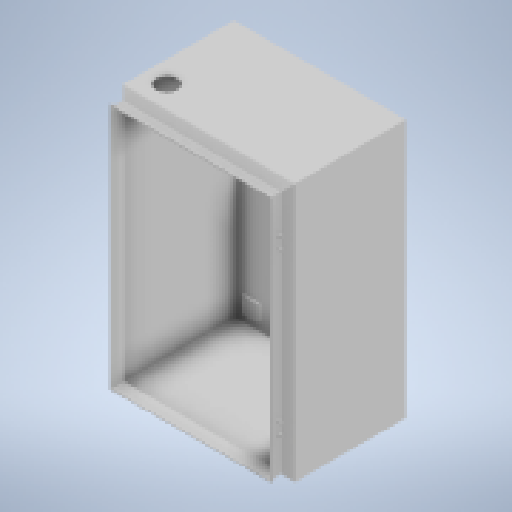
# Autodesk Inventor part: 1301.000_1_(1)
Saved by Autodesk Inventor 2025.2 (Build 292293000, 293)
## iProperties
Category: PARTsolutions
Company: RITTAL
Created: 2025-05-02
Part Number: 1301.000_1_(1)
Material: Generic
Catalog Web Link: www.cadenas.de
Description: Gehaeuse KX EB Edelstahl-Gehaeuse KX EB Edelstahl
Vendor: RITTAL
Document SubType Name: Modeling
Designer: psAdmin
Manufacturer: RITTAL
Mass: 264.521 g
Surface Area: 4243.67 cm^2
Volume: 264.521 cm^3
Density: 1 g/cm^3
Appearance: PSOLRGB-175-175-175
PSOL_IDENT_0: {$CADENAS_DATA/23d-libs/rittal/schaltschranksys/edelstahl/kleingehause/parts_eb_edel_2_0/gehaeuse_kx
PSOL_IDENT_1: _eb_edel_new.prj},199 {VTYP=3D},{NB=1301.000_1_(1)},{LINA=1301.000_1_(1)},{NN=Gehaeuse KX EB Edelsta
PSOL_IDENT_2: hl},{DATE=28.04.2025 21:10:48},{GEOMDATE=11.04.2025 11:21:29},{VERSION=},{LINEID=690},{WBVAR=DETAIL}
PSOL_IDENT_3: ,{WBNUMERIC=DETAIL}  {NB=1301.000_1_(1)},{LINA=1301.000_1_(1)},{KT=DUMMY},{BEST=1301.000},{S=1.25},{
PSOL_IDENT_4: DETAIL=1},{B1=200},{H1=300},{T1=152.750},{B2=160.000},{B3=187},{L=133},{L1=75},{N=6},{H2=260},{T=155
PSOL_IDENT_5: .000},{GEW=3,889},{T2=130.000},{CNSETIM80=EC000261},{CNSETIM90=EC000261},{CNSECLASS60=27-18-01-01},{
PSOL_IDENT_6: CNSECLASS80=27-18-01-01},{UNSPSC=31-26-15-02}
NB: 1301.000_1_(1)
NN: Gehaeuse KX EB Edelstahl
NT: Gehaeuse KX EB Edelstahl
NBSYN: $BEST._1_($DETAIL.)
LINA: 1301.000_1_(1)
CATALOG: Rittal
BEST: 1301.000
S: 1.25
DETAIL: hoch
B1: 200
H1: 300
T1: 152.75
B2: 160
B3: 187
L: 133
L1: 75
N: 6
H2: 260
T: 155
GEW: 3,889
T2: 130
CNSETIM80: EC000261
CNSETIM90: EC000261
CNSECLASS60: 27-18-01-01
CNSECLASS80: 27-18-01-01
UNSPSC: 31-26-15-02
SUPPLIER: RITTAL
ARTICLENO: 1301.000_1_(1)
BOMINFO: 1301.000_1_(1)
CREATOR: CADENAS GmbH
Title: 1301.000_1_(1)
Author: Cadenas PARTsolutions
Comments: Gehaeuse KX EB Edelstahl
Autodesk Inventor part; units mm, degrees
(part 1 of 2)
ref_plane "YZ Plane" through (0, 0, 0) normal (1, 0, 0) x (0, 1, 0)
ref_plane "XZ Plane" through (0, 0, 0) normal (0, 1, 0) x (-1, 0, 0)
ref_plane "XY Plane" through (0, 0, 0) normal (0, 0, 1) x (1, 0, 0)
sketch "Skizze_2" plane through (0, 0, 0) normal (1, 0, 0) x (0, 0, -1)
  line L0 (-75.4448, -142.2749) -> (-75.1213, -143.4823)
  line L1 (-75.1213, -143.4823) -> (-69.0017, -141.8426)
  arc A0 (-68.6782, -141.8) -> (-69.0017, -141.8426) centre (-68.6782, -143.05) ccw
  line L2 (-68.6782, -141.8) -> (-62.8605, -141.8)
  arc A1 (-61.9767, -142.1661) -> (-62.8605, -141.8) centre (-62.8605, -143.05) ccw
  line L3 (-61.9767, -142.1661) -> (-54.875, -149.2678)
  arc A2 (-54.875, -149.2678) -> (-53.1072, -150) centre (-53.1072, -147.5) ccw
  line L4 (-53.1072, -150) -> (76.375, -150)
  line L5 (76.375, -150) -> (76.375, 150)
  line L6 (76.375, 150) -> (-53.1072, 150)
  arc A3 (-53.1072, 150) -> (-54.875, 149.2678) centre (-53.1072, 147.5) ccw
  line L7 (-54.875, 149.2678) -> (-61.9767, 142.1661)
  arc A4 (-62.8605, 141.8) -> (-61.9767, 142.1661) centre (-62.8605, 143.05) ccw
  line L8 (-62.8605, 141.8) -> (-68.6782, 141.8)
  arc A5 (-69.0017, 141.8426) -> (-68.6782, 141.8) centre (-68.6782, 143.05) ccw
  line L9 (-69.0017, 141.8426) -> (-75.1213, 143.4823)
  line L10 (-75.1213, 143.4823) -> (-75.4448, 142.2749)
  line L11 (-75.4448, 142.2749) -> (-69.3252, 140.6352)
  arc A6 (-69.3252, 140.6352) -> (-68.6782, 140.55) centre (-68.6782, 143.05) ccw
  line L12 (-68.6782, 140.55) -> (-62.8605, 140.55)
  arc A7 (-62.8605, 140.55) -> (-61.0928, 141.2822) centre (-62.8605, 143.05) ccw
  line L13 (-61.0928, 141.2822) -> (-53.9911, 148.3839)
  arc A8 (-53.1072, 148.75) -> (-53.9911, 148.3839) centre (-53.1072, 147.5) ccw
  line L14 (-53.1072, 148.75) -> (73.875, 148.75)
  arc A9 (75.125, 147.5) -> (73.875, 148.75) centre (73.875, 147.5) ccw
  line L15 (75.125, 147.5) -> (75.125, -147.5)
  arc A10 (73.875, -148.75) -> (75.125, -147.5) centre (73.875, -147.5) ccw
  line L16 (73.875, -148.75) -> (-53.1072, -148.75)
  arc A11 (-53.9911, -148.3839) -> (-53.1072, -148.75) centre (-53.1072, -147.5) ccw
  line L17 (-53.9911, -148.3839) -> (-61.0928, -141.2822)
  arc A12 (-61.0928, -141.2822) -> (-62.8605, -140.55) centre (-62.8605, -143.05) ccw
  line L18 (-62.8605, -140.55) -> (-68.6782, -140.55)
  arc A13 (-68.6782, -140.55) -> (-69.3252, -140.6352) centre (-68.6782, -143.05) ccw
  line L19 (-69.3252, -140.6352) -> (-75.4448, -142.2749)
  constraints: 40 end point, 28 point on circle, 14 centre point
extrude "Extrusion1" add sketch "Skizze_2" along normal mid plane 200
sketch "Sketch_1" plane through (0, 0, 0) normal (0, 1, 0) x (-1, 0, 0)
  line L0 (100, -76.375) -> (100, 53.1072)
  arc A0 (100, 53.1072) -> (99.2678, 54.875) centre (97.5, 53.1072) ccw
  line L1 (99.2678, 54.875) -> (92.1661, 61.9767)
  arc A1 (91.8, 62.8605) -> (92.1661, 61.9767) centre (93.05, 62.8605) ccw
  line L2 (91.8, 62.8605) -> (91.8, 68.6782)
  arc A2 (91.8426, 69.0017) -> (91.8, 68.6782) centre (93.05, 68.6782) ccw
  line L3 (91.8426, 69.0017) -> (93.4823, 75.1213)
  line L4 (93.4823, 75.1213) -> (92.2749, 75.4448)
  line L5 (92.2749, 75.4448) -> (90.6352, 69.3252)
  arc A3 (90.6352, 69.3252) -> (90.55, 68.6782) centre (93.05, 68.6782) ccw
  line L6 (90.55, 68.6782) -> (90.55, 62.8605)
  arc A4 (90.55, 62.8605) -> (91.2822, 61.0928) centre (93.05, 62.8605) ccw
  line L7 (91.2822, 61.0928) -> (98.3839, 53.9911)
  arc A5 (98.75, 53.1072) -> (98.3839, 53.9911) centre (97.5, 53.1072) ccw
  line L8 (98.75, 53.1072) -> (98.75, -73.875)
  arc A6 (97.5, -75.125) -> (98.75, -73.875) centre (97.5, -73.875) ccw
  line L9 (97.5, -75.125) -> (-97.5, -75.125)
  arc A7 (-98.75, -73.875) -> (-97.5, -75.125) centre (-97.5, -73.875) ccw
  line L10 (-98.75, -73.875) -> (-98.75, 53.1072)
  arc A8 (-98.3839, 53.9911) -> (-98.75, 53.1072) centre (-97.5, 53.1072) ccw
  line L11 (-98.3839, 53.9911) -> (-91.2822, 61.0928)
  arc A9 (-91.2822, 61.0928) -> (-90.55, 62.8605) centre (-93.05, 62.8605) ccw
  line L12 (-90.55, 62.8605) -> (-90.55, 68.6782)
  arc A10 (-90.55, 68.6782) -> (-90.6352, 69.3252) centre (-93.05, 68.6782) ccw
  line L13 (-90.6352, 69.3252) -> (-92.2749, 75.4448)
  line L14 (-92.2749, 75.4448) -> (-93.4823, 75.1213)
  line L15 (-93.4823, 75.1213) -> (-91.8426, 69.0017)
  arc A11 (-91.8, 68.6782) -> (-91.8426, 69.0017) centre (-93.05, 68.6782) ccw
  line L16 (-91.8, 68.6782) -> (-91.8, 62.8605)
  arc A12 (-92.1661, 61.9767) -> (-91.8, 62.8605) centre (-93.05, 62.8605) ccw
  line L17 (-92.1661, 61.9767) -> (-99.2678, 54.875)
  arc A13 (-99.2678, 54.875) -> (-100, 53.1072) centre (-97.5, 53.1072) ccw
  line L18 (-100, 53.1072) -> (-100, -76.375)
  line L19 (-100, -76.375) -> (100, -76.375)
  constraints: 40 end point, 28 point on circle, 14 centre point
extrude "Extrusion2" add sketch "Sketch_1" along normal mid plane 300
sketch "Sketch_37" plane through (0, 0, 0) normal (1, 0, 0) x (0, 0, -1)
  line L0 (-86.375, -160) -> (86.375, -160)
  line L1 (86.375, -160) -> (86.375, 160)
  line L2 (86.375, 160) -> (-86.375, 160)
  line L3 (-86.375, 160) -> (-86.375, -160)
  line L4 (-75.4448, -142.2749) -> (-75.1213, -143.4823)
  line L5 (-75.1213, -143.4823) -> (-69.0017, -141.8426)
  arc A0 (-68.6782, -141.8) -> (-69.0017, -141.8426) centre (-68.6782, -143.05) ccw
  line L6 (-68.6782, -141.8) -> (-62.8605, -141.8)
  arc A1 (-61.9767, -142.1661) -> (-62.8605, -141.8) centre (-62.8605, -143.05) ccw
  line L7 (-61.9767, -142.1661) -> (-54.875, -149.2678)
  arc A2 (-54.875, -149.2678) -> (-53.1072, -150) centre (-53.1072, -147.5) ccw
  line L8 (-53.1072, -150) -> (73.875, -150)
  arc A3 (73.875, -150) -> (76.375, -147.5) centre (73.875, -147.5) ccw
  line L9 (76.375, -147.5) -> (76.375, 147.5)
  arc A4 (76.375, 147.5) -> (73.875, 150) centre (73.875, 147.5) ccw
  line L10 (73.875, 150) -> (-53.1072, 150)
  arc A5 (-53.1072, 150) -> (-54.875, 149.2678) centre (-53.1072, 147.5) ccw
  line L11 (-54.875, 149.2678) -> (-61.9767, 142.1661)
  arc A6 (-62.8605, 141.8) -> (-61.9767, 142.1661) centre (-62.8605, 143.05) ccw
  line L12 (-62.8605, 141.8) -> (-68.6782, 141.8)
  arc A7 (-69.0017, 141.8426) -> (-68.6782, 141.8) centre (-68.6782, 143.05) ccw
  line L13 (-69.0017, 141.8426) -> (-75.1213, 143.4823)
  line L14 (-75.1213, 143.4823) -> (-75.4448, 142.2749)
  line L15 (-75.4448, 142.2749) -> (-75.4448, -142.2749)
  constraints: 32 end point, 16 point on circle, 8 centre point
extrude "Extrusion3" cut sketch "Sketch_37" along normal mid plane 200
sketch "Sketch_38" plane through (0, 0, 0) normal (0, 1, 0) x (-1, 0, 0)
  line L0 (110, 86.375) -> (-110, 86.375)
  line L1 (-110, 86.375) -> (-110, -86.375)
  line L2 (-110, -86.375) -> (110, -86.375)
  line L3 (110, -86.375) -> (110, 86.375)
  line L4 (100, -73.875) -> (100, 53.1072)
  arc A0 (100, 53.1072) -> (99.2678, 54.875) centre (97.5, 53.1072) ccw
  line L5 (99.2678, 54.875) -> (92.1661, 61.9767)
  arc A1 (91.8, 62.8605) -> (92.1661, 61.9767) centre (93.05, 62.8605) ccw
  line L6 (91.8, 62.8605) -> (91.8, 68.6782)
  arc A2 (91.8426, 69.0017) -> (91.8, 68.6782) centre (93.05, 68.6782) ccw
  line L7 (91.8426, 69.0017) -> (93.4823, 75.1213)
  line L8 (93.4823, 75.1213) -> (92.2749, 75.4448)
  line L9 (92.2749, 75.4448) -> (-92.2749, 75.4448)
  line L10 (-92.2749, 75.4448) -> (-93.4823, 75.1213)
  line L11 (-93.4823, 75.1213) -> (-91.8426, 69.0017)
  arc A3 (-91.8, 68.6782) -> (-91.8426, 69.0017) centre (-93.05, 68.6782) ccw
  line L12 (-91.8, 68.6782) -> (-91.8, 62.8605)
  arc A4 (-92.1661, 61.9767) -> (-91.8, 62.8605) centre (-93.05, 62.8605) ccw
  line L13 (-92.1661, 61.9767) -> (-99.2678, 54.875)
  arc A5 (-99.2678, 54.875) -> (-100, 53.1072) centre (-97.5, 53.1072) ccw
  line L14 (-100, 53.1072) -> (-100, -73.875)
  arc A6 (-100, -73.875) -> (-97.5, -76.375) centre (-97.5, -73.875) ccw
  line L15 (-97.5, -76.375) -> (97.5, -76.375)
  arc A7 (97.5, -76.375) -> (100, -73.875) centre (97.5, -73.875) ccw
  constraints: 32 end point, 16 point on circle, 8 centre point
extrude "Extrusion4" cut sketch "Sketch_38" along normal mid plane 300
sketch "Sketch_2" plane through (0, 0, -76.375) normal (0, 0, 1) x (1, 0, 0)
  line L0 (67.5, 142.5) -> (67.5, 117.5)
  line L1 (67.5, 117.5) -> (92.5, 117.5)
  line L2 (92.5, 117.5) -> (92.5, 142.5)
  line L3 (92.5, 142.5) -> (67.5, 142.5)
  constraints: 8 end point
extrude "Extrusion5" cut sketch "Sketch_2" along normal blind 3.25
sketch "Sketch_9" plane through (0, 0, -76.375) normal (0, 0, 1) x (1, 0, 0)
  line L0 (-92.5, 142.5) -> (-92.5, 117.5)
  line L1 (-92.5, 117.5) -> (-67.5, 117.5)
  line L2 (-67.5, 117.5) -> (-67.5, 142.5)
  line L3 (-67.5, 142.5) -> (-92.5, 142.5)
  constraints: 8 end point
extrude "Extrusion6" cut sketch "Sketch_9" along normal blind 3.25
sketch "Sketch_10" plane through (0, 0, -76.375) normal (0, 0, 1) x (1, 0, 0)
  line L0 (67.5, -117.5) -> (67.5, -142.5)
  line L1 (67.5, -142.5) -> (92.5, -142.5)
  line L2 (92.5, -142.5) -> (92.5, -117.5)
  line L3 (92.5, -117.5) -> (67.5, -117.5)
  constraints: 8 end point
extrude "Extrusion7" cut sketch "Sketch_10" along normal blind 3.25
sketch "Sketch_11" plane through (0, 0, -76.375) normal (0, 0, 1) x (1, 0, 0)
  line L0 (-92.5, -117.5) -> (-92.5, -142.5)
  line L1 (-92.5, -142.5) -> (-67.5, -142.5)
  line L2 (-67.5, -142.5) -> (-67.5, -117.5)
  line L3 (-67.5, -117.5) -> (-92.5, -117.5)
  constraints: 8 end point
extrude "Extrusion8" cut sketch "Sketch_11" along normal blind 3.25
sketch "Sketch_30" plane through (0, 130, 0) normal (0, 1, 0) x (1, 0, 0)
  line L0 (66.5, 75.125) -> (69.0034, 75.125)
  arc A0 (69.2528, 74.9917) -> (69.0034, 75.125) centre (69.0034, 74.825) ccw
  line L1 (69.2528, 74.9917) -> (70.0546, 73.7917)
  arc A1 (70.0546, 73.7917) -> (71.3018, 73.125) centre (71.3018, 74.625) ccw
  line L2 (71.3018, 73.125) -> (88.6982, 73.125)
  arc A2 (88.6982, 73.125) -> (89.9454, 73.7917) centre (88.6982, 74.625) ccw
  line L3 (89.9454, 73.7917) -> (90.7472, 74.9917)
  arc A3 (90.9966, 75.125) -> (90.7472, 74.9917) centre (90.9966, 74.825) ccw
  line L4 (90.9966, 75.125) -> (93.5, 75.125)
  line L5 (93.5, 75.125) -> (93.5, 76.375)
  line L6 (93.5, 76.375) -> (90.9699, 76.375)
  arc A4 (90.9699, 76.375) -> (89.7227, 75.7083) centre (90.9699, 74.875) ccw
  line L7 (89.7227, 75.7083) -> (88.9209, 74.5083)
  arc A5 (88.6715, 74.375) -> (88.9209, 74.5083) centre (88.6715, 74.675) ccw
  line L8 (88.6715, 74.375) -> (71.3285, 74.375)
  arc A6 (71.0791, 74.5083) -> (71.3285, 74.375) centre (71.3285, 74.675) ccw
  line L9 (71.0791, 74.5083) -> (70.2773, 75.7083)
  arc A7 (70.2773, 75.7083) -> (69.0301, 76.375) centre (69.0301, 74.875) ccw
  line L10 (69.0301, 76.375) -> (66.5, 76.375)
  line L11 (66.5, 76.375) -> (66.5, 75.125)
  constraints: 24 end point, 16 point on circle, 8 centre point
extrude "Extrusion9" add sketch "Sketch_30" along normal mid plane 15.297
sketch "Sketch_31" plane through (0, 130, 0) normal (0, 1, 0) x (1, 0, 0)
  line L0 (-93.5, 75.125) -> (-90.9966, 75.125)
  arc A0 (-90.7472, 74.9917) -> (-90.9966, 75.125) centre (-90.9966, 74.825) ccw
  line L1 (-90.7472, 74.9917) -> (-89.9454, 73.7917)
  arc A1 (-89.9454, 73.7917) -> (-88.6982, 73.125) centre (-88.6982, 74.625) ccw
  line L2 (-88.6982, 73.125) -> (-71.3018, 73.125)
  arc A2 (-71.3018, 73.125) -> (-70.0546, 73.7917) centre (-71.3018, 74.625) ccw
  line L3 (-70.0546, 73.7917) -> (-69.2528, 74.9917)
  arc A3 (-69.0034, 75.125) -> (-69.2528, 74.9917) centre (-69.0034, 74.825) ccw
  line L4 (-69.0034, 75.125) -> (-66.5, 75.125)
  line L5 (-66.5, 75.125) -> (-66.5, 76.375)
  line L6 (-66.5, 76.375) -> (-69.0301, 76.375)
  arc A4 (-69.0301, 76.375) -> (-70.2773, 75.7083) centre (-69.0301, 74.875) ccw
  line L7 (-70.2773, 75.7083) -> (-71.0791, 74.5083)
  arc A5 (-71.3285, 74.375) -> (-71.0791, 74.5083) centre (-71.3285, 74.675) ccw
  line L8 (-71.3285, 74.375) -> (-88.6715, 74.375)
  arc A6 (-88.9209, 74.5083) -> (-88.6715, 74.375) centre (-88.6715, 74.675) ccw
  line L9 (-88.9209, 74.5083) -> (-89.7227, 75.7083)
  arc A7 (-89.7227, 75.7083) -> (-90.9699, 76.375) centre (-90.9699, 74.875) ccw
  line L10 (-90.9699, 76.375) -> (-93.5, 76.375)
  line L11 (-93.5, 76.375) -> (-93.5, 75.125)
  constraints: 24 end point, 16 point on circle, 8 centre point
extrude "Extrusion10" add sketch "Sketch_31" along normal mid plane 15.297
sketch "Sketch_32" plane through (0, -130, 0) normal (0, 1, 0) x (1, 0, 0)
  line L0 (66.5, 75.125) -> (69.0034, 75.125)
  arc A0 (69.2528, 74.9917) -> (69.0034, 75.125) centre (69.0034, 74.825) ccw
  line L1 (69.2528, 74.9917) -> (70.0546, 73.7917)
  arc A1 (70.0546, 73.7917) -> (71.3018, 73.125) centre (71.3018, 74.625) ccw
  line L2 (71.3018, 73.125) -> (88.6982, 73.125)
  arc A2 (88.6982, 73.125) -> (89.9454, 73.7917) centre (88.6982, 74.625) ccw
  line L3 (89.9454, 73.7917) -> (90.7472, 74.9917)
  arc A3 (90.9966, 75.125) -> (90.7472, 74.9917) centre (90.9966, 74.825) ccw
  line L4 (90.9966, 75.125) -> (93.5, 75.125)
  line L5 (93.5, 75.125) -> (93.5, 76.375)
  line L6 (93.5, 76.375) -> (90.9699, 76.375)
  arc A4 (90.9699, 76.375) -> (89.7227, 75.7083) centre (90.9699, 74.875) ccw
  line L7 (89.7227, 75.7083) -> (88.9209, 74.5083)
  arc A5 (88.6715, 74.375) -> (88.9209, 74.5083) centre (88.6715, 74.675) ccw
  line L8 (88.6715, 74.375) -> (71.3285, 74.375)
  arc A6 (71.0791, 74.5083) -> (71.3285, 74.375) centre (71.3285, 74.675) ccw
  line L9 (71.0791, 74.5083) -> (70.2773, 75.7083)
  arc A7 (70.2773, 75.7083) -> (69.0301, 76.375) centre (69.0301, 74.875) ccw
  line L10 (69.0301, 76.375) -> (66.5, 76.375)
  line L11 (66.5, 76.375) -> (66.5, 75.125)
  constraints: 24 end point, 16 point on circle, 8 centre point
extrude "Extrusion11" add sketch "Sketch_32" along normal mid plane 15.297
sketch "Sketch_33" plane through (0, -130, 0) normal (0, 1, 0) x (1, 0, 0)
  line L0 (-93.5, 75.125) -> (-90.9966, 75.125)
  arc A0 (-90.7472, 74.9917) -> (-90.9966, 75.125) centre (-90.9966, 74.825) ccw
  line L1 (-90.7472, 74.9917) -> (-89.9454, 73.7917)
  arc A1 (-89.9454, 73.7917) -> (-88.6982, 73.125) centre (-88.6982, 74.625) ccw
  line L2 (-88.6982, 73.125) -> (-71.3018, 73.125)
  arc A2 (-71.3018, 73.125) -> (-70.0546, 73.7917) centre (-71.3018, 74.625) ccw
  line L3 (-70.0546, 73.7917) -> (-69.2528, 74.9917)
  arc A3 (-69.0034, 75.125) -> (-69.2528, 74.9917) centre (-69.0034, 74.825) ccw
  line L4 (-69.0034, 75.125) -> (-66.5, 75.125)
  line L5 (-66.5, 75.125) -> (-66.5, 76.375)
  line L6 (-66.5, 76.375) -> (-69.0301, 76.375)
  arc A4 (-69.0301, 76.375) -> (-70.2773, 75.7083) centre (-69.0301, 74.875) ccw
  line L7 (-70.2773, 75.7083) -> (-71.0791, 74.5083)
  arc A5 (-71.3285, 74.375) -> (-71.0791, 74.5083) centre (-71.3285, 74.675) ccw
  line L8 (-71.3285, 74.375) -> (-88.6715, 74.375)
  arc A6 (-88.9209, 74.5083) -> (-88.6715, 74.375) centre (-88.6715, 74.675) ccw
  line L9 (-88.9209, 74.5083) -> (-89.7227, 75.7083)
  arc A7 (-89.7227, 75.7083) -> (-90.9699, 76.375) centre (-90.9699, 74.875) ccw
  line L10 (-90.9699, 76.375) -> (-93.5, 76.375)
  line L11 (-93.5, 76.375) -> (-93.5, 75.125)
  constraints: 24 end point, 16 point on circle, 8 centre point
extrude "Extrusion12" add sketch "Sketch_33" along normal mid plane 15.297
sketch "Sketch_43" plane through (-80, 0, 0) normal (1, 0, 0) x (0, 0, -1)
  line L0 (73.125, -121.3018) -> (73.125, -138.6982)
  arc A0 (73.125, -138.6982) -> (73.7917, -139.9454) centre (74.625, -138.6982) ccw
  line L1 (73.7917, -139.9454) -> (74.9917, -140.7472)
  arc A1 (75.125, -140.9966) -> (74.9917, -140.7472) centre (74.825, -140.9966) ccw
  line L2 (75.125, -140.9966) -> (75.125, -143.5)
  line L3 (75.125, -143.5) -> (76.375, -143.5)
  line L4 (76.375, -143.5) -> (76.375, -140.9699)
  arc A2 (76.375, -140.9699) -> (75.7083, -139.7227) centre (74.875, -140.9699) ccw
  line L5 (75.7083, -139.7227) -> (74.5083, -138.9209)
  arc A3 (74.375, -138.6715) -> (74.5083, -138.9209) centre (74.675, -138.6715) ccw
  line L6 (74.375, -138.6715) -> (74.375, -121.3285)
  arc A4 (74.5083, -121.0791) -> (74.375, -121.3285) centre (74.675, -121.3285) ccw
  line L7 (74.5083, -121.0791) -> (75.7083, -120.2773)
  arc A5 (75.7083, -120.2773) -> (76.375, -119.0301) centre (74.875, -119.0301) ccw
  line L8 (76.375, -119.0301) -> (76.375, -116.5)
  line L9 (76.375, -116.5) -> (75.125, -116.5)
  line L10 (75.125, -116.5) -> (75.125, -119.0034)
  arc A6 (74.9917, -119.2528) -> (75.125, -119.0034) centre (74.825, -119.0034) ccw
  line L11 (74.9917, -119.2528) -> (73.7917, -120.0546)
  arc A7 (73.7917, -120.0546) -> (73.125, -121.3018) centre (74.625, -121.3018) ccw
  constraints: 24 end point, 16 point on circle, 8 centre point
extrude "Extrusion13" add sketch "Sketch_43" along normal mid plane 15.297
sketch "Sketch_44" plane through (80, 0, 0) normal (1, 0, 0) x (0, 0, -1)
  line L0 (73.125, -121.3018) -> (73.125, -138.6982)
  arc A0 (73.125, -138.6982) -> (73.7917, -139.9454) centre (74.625, -138.6982) ccw
  line L1 (73.7917, -139.9454) -> (74.9917, -140.7472)
  arc A1 (75.125, -140.9966) -> (74.9917, -140.7472) centre (74.825, -140.9966) ccw
  line L2 (75.125, -140.9966) -> (75.125, -143.5)
  line L3 (75.125, -143.5) -> (76.375, -143.5)
  line L4 (76.375, -143.5) -> (76.375, -140.9699)
  arc A2 (76.375, -140.9699) -> (75.7083, -139.7227) centre (74.875, -140.9699) ccw
  line L5 (75.7083, -139.7227) -> (74.5083, -138.9209)
  arc A3 (74.375, -138.6715) -> (74.5083, -138.9209) centre (74.675, -138.6715) ccw
  line L6 (74.375, -138.6715) -> (74.375, -121.3285)
  arc A4 (74.5083, -121.0791) -> (74.375, -121.3285) centre (74.675, -121.3285) ccw
  line L7 (74.5083, -121.0791) -> (75.7083, -120.2773)
  arc A5 (75.7083, -120.2773) -> (76.375, -119.0301) centre (74.875, -119.0301) ccw
  line L8 (76.375, -119.0301) -> (76.375, -116.5)
  line L9 (76.375, -116.5) -> (75.125, -116.5)
  line L10 (75.125, -116.5) -> (75.125, -119.0034)
  arc A6 (74.9917, -119.2528) -> (75.125, -119.0034) centre (74.825, -119.0034) ccw
  line L11 (74.9917, -119.2528) -> (73.7917, -120.0546)
  arc A7 (73.7917, -120.0546) -> (73.125, -121.3018) centre (74.625, -121.3018) ccw
  constraints: 24 end point, 16 point on circle, 8 centre point
extrude "Extrusion14" add sketch "Sketch_44" along normal mid plane 15.297
sketch "Sketch_45" plane through (-80, 0, 0) normal (1, 0, 0) x (0, 0, -1)
  arc A0 (73.125, 121.3018) -> (73.7917, 120.0546) centre (74.625, 121.3018) ccw
  line L0 (73.7917, 120.0546) -> (74.9917, 119.2528)
  arc A1 (75.125, 119.0034) -> (74.9917, 119.2528) centre (74.825, 119.0034) ccw
  line L1 (75.125, 119.0034) -> (75.125, 116.5)
  line L2 (75.125, 116.5) -> (76.375, 116.5)
  line L3 (76.375, 116.5) -> (76.375, 119.0301)
  arc A2 (76.375, 119.0301) -> (75.7083, 120.2773) centre (74.875, 119.0301) ccw
  line L4 (75.7083, 120.2773) -> (74.5083, 121.0791)
  arc A3 (74.375, 121.3285) -> (74.5083, 121.0791) centre (74.675, 121.3285) ccw
  line L5 (74.375, 121.3285) -> (74.375, 138.6715)
  arc A4 (74.5083, 138.9209) -> (74.375, 138.6715) centre (74.675, 138.6715) ccw
  line L6 (74.5083, 138.9209) -> (75.7083, 139.7227)
  arc A5 (75.7083, 139.7227) -> (76.375, 140.9699) centre (74.875, 140.9699) ccw
  line L7 (76.375, 140.9699) -> (76.375, 143.5)
  line L8 (76.375, 143.5) -> (75.125, 143.5)
  line L9 (75.125, 143.5) -> (75.125, 140.9966)
  arc A6 (74.9917, 140.7472) -> (75.125, 140.9966) centre (74.825, 140.9966) ccw
  line L10 (74.9917, 140.7472) -> (73.7917, 139.9454)
  arc A7 (73.7917, 139.9454) -> (73.125, 138.6982) centre (74.625, 138.6982) ccw
  line L11 (73.125, 138.6982) -> (73.125, 121.3018)
  constraints: 24 end point, 16 point on circle, 8 centre point
extrude "Extrusion15" add sketch "Sketch_45" along normal mid plane 15.297
sketch "Sketch_46" plane through (80, 0, 0) normal (1, 0, 0) x (0, 0, -1)
  arc A0 (73.125, 121.3018) -> (73.7917, 120.0546) centre (74.625, 121.3018) ccw
  line L0 (73.7917, 120.0546) -> (74.9917, 119.2528)
  arc A1 (75.125, 119.0034) -> (74.9917, 119.2528) centre (74.825, 119.0034) ccw
  line L1 (75.125, 119.0034) -> (75.125, 116.5)
  line L2 (75.125, 116.5) -> (76.375, 116.5)
  line L3 (76.375, 116.5) -> (76.375, 119.0301)
  arc A2 (76.375, 119.0301) -> (75.7083, 120.2773) centre (74.875, 119.0301) ccw
  line L4 (75.7083, 120.2773) -> (74.5083, 121.0791)
  arc A3 (74.375, 121.3285) -> (74.5083, 121.0791) centre (74.675, 121.3285) ccw
  line L5 (74.375, 121.3285) -> (74.375, 138.6715)
  arc A4 (74.5083, 138.9209) -> (74.375, 138.6715) centre (74.675, 138.6715) ccw
  line L6 (74.5083, 138.9209) -> (75.7083, 139.7227)
  arc A5 (75.7083, 139.7227) -> (76.375, 140.9699) centre (74.875, 140.9699) ccw
  line L7 (76.375, 140.9699) -> (76.375, 143.5)
  line L8 (76.375, 143.5) -> (75.125, 143.5)
  line L9 (75.125, 143.5) -> (75.125, 140.9966)
  arc A6 (74.9917, 140.7472) -> (75.125, 140.9966) centre (74.825, 140.9966) ccw
  line L10 (74.9917, 140.7472) -> (73.7917, 139.9454)
  arc A7 (73.7917, 139.9454) -> (73.125, 138.6982) centre (74.625, 138.6982) ccw
  line L11 (73.125, 138.6982) -> (73.125, 121.3018)
  constraints: 24 end point, 16 point on circle, 8 centre point
extrude "Extrusion16" add sketch "Sketch_46" along normal mid plane 15.297
sketch "Sketch_47" plane through (0, -122.3515, 0) normal (0, 1, 0) x (1, 0, 0)
  line L0 (72.3515, 74.375) -> (72.3515, 73.125)
  line L1 (72.3515, 73.125) -> (71.3018, 73.125)
  arc A0 (70.0546, 73.7917) -> (71.3018, 73.125) centre (71.3018, 74.625) ccw
  line L2 (70.0546, 73.7917) -> (69.2528, 74.9917)
  arc A1 (69.2528, 74.9917) -> (69.0034, 75.125) centre (69.0034, 74.825) ccw
  line L3 (69.0034, 75.125) -> (60.5, 75.125)
  line L4 (60.5, 75.125) -> (60.5, 76.375)
  line L5 (60.5, 76.375) -> (69.0301, 76.375)
  arc A2 (70.2773, 75.7083) -> (69.0301, 76.375) centre (69.0301, 74.875) ccw
  line L6 (70.2773, 75.7083) -> (71.0791, 74.5083)
  arc A3 (71.0791, 74.5083) -> (71.3285, 74.375) centre (71.3285, 74.675) ccw
  line L7 (71.3285, 74.375) -> (72.3515, 74.375)
  line L8 (72.3515, 74.375) -> (72.3515, 73.125)
  constraints: 18 end point, 8 point on circle, 4 centre point
revolve "Revolution1" add sketch "Sketch_47" angle 90 about axis through (72.3515, -122.3515, -74.375) along (0, 0, -1)
sketch "Sketch_48" plane through (0, -122.3515, 0) normal (0, 1, 0) x (1, 0, 0)
  line L0 (87.6485, 73.125) -> (87.6485, 74.375)
  line L1 (87.6485, 74.375) -> (88.6715, 74.375)
  arc A0 (88.6715, 74.375) -> (88.9209, 74.5083) centre (88.6715, 74.675) ccw
  line L2 (88.9209, 74.5083) -> (89.7227, 75.7083)
  arc A1 (90.9699, 76.375) -> (89.7227, 75.7083) centre (90.9699, 74.875) ccw
  line L3 (90.9699, 76.375) -> (95.5, 76.375)
  line L4 (95.5, 76.375) -> (95.5, 75.125)
  line L5 (95.5, 75.125) -> (90.9966, 75.125)
  arc A2 (90.9966, 75.125) -> (90.7472, 74.9917) centre (90.9966, 74.825) ccw
  line L6 (90.7472, 74.9917) -> (89.9454, 73.7917)
  arc A3 (88.6982, 73.125) -> (89.9454, 73.7917) centre (88.6982, 74.625) ccw
  line L7 (88.6982, 73.125) -> (87.6485, 73.125)
  line L8 (87.6485, 73.125) -> (87.6485, 74.375)
  constraints: 18 end point, 8 point on circle, 4 centre point
revolve "Revolution2" add sketch "Sketch_48" angle 90 about axis through (87.6485, -122.3515, -73.125) along (0, 0, 1)
sketch "Sketch_49" plane through (0, -122.3515, 0) normal (0, 1, 0) x (1, 0, 0)
  line L0 (-72.3515, 73.125) -> (-72.3515, 74.375)
  line L1 (-72.3515, 74.375) -> (-71.3285, 74.375)
  arc A0 (-71.3285, 74.375) -> (-71.0791, 74.5083) centre (-71.3285, 74.675) ccw
  line L2 (-71.0791, 74.5083) -> (-70.2773, 75.7083)
  arc A1 (-69.0301, 76.375) -> (-70.2773, 75.7083) centre (-69.0301, 74.875) ccw
  line L3 (-69.0301, 76.375) -> (-64.5, 76.375)
  line L4 (-64.5, 76.375) -> (-64.5, 75.125)
  line L5 (-64.5, 75.125) -> (-69.0034, 75.125)
  arc A2 (-69.0034, 75.125) -> (-69.2528, 74.9917) centre (-69.0034, 74.825) ccw
  line L6 (-69.2528, 74.9917) -> (-70.0546, 73.7917)
  arc A3 (-71.3018, 73.125) -> (-70.0546, 73.7917) centre (-71.3018, 74.625) ccw
  line L7 (-71.3018, 73.125) -> (-72.3515, 73.125)
  line L8 (-72.3515, 73.125) -> (-72.3515, 74.375)
  constraints: 18 end point, 8 point on circle, 4 centre point
revolve "Revolution3" add sketch "Sketch_49" angle 90 about axis through (-72.3515, -122.3515, -73.125) along (0, 0, 1)
sketch "Sketch_50" plane through (0, -122.3515, 0) normal (0, 1, 0) x (1, 0, 0)
  line L0 (-87.6485, 74.375) -> (-87.6485, 73.125)
  line L1 (-87.6485, 73.125) -> (-88.6982, 73.125)
  arc A0 (-89.9454, 73.7917) -> (-88.6982, 73.125) centre (-88.6982, 74.625) ccw
  line L2 (-89.9454, 73.7917) -> (-90.7472, 74.9917)
  arc A1 (-90.7472, 74.9917) -> (-90.9966, 75.125) centre (-90.9966, 74.825) ccw
  line L3 (-90.9966, 75.125) -> (-95.5, 75.125)
  line L4 (-95.5, 75.125) -> (-95.5, 76.375)
  line L5 (-95.5, 76.375) -> (-90.9699, 76.375)
  arc A2 (-89.7227, 75.7083) -> (-90.9699, 76.375) centre (-90.9699, 74.875) ccw
  line L6 (-89.7227, 75.7083) -> (-88.9209, 74.5083)
  arc A3 (-88.9209, 74.5083) -> (-88.6715, 74.375) centre (-88.6715, 74.675) ccw
  line L7 (-88.6715, 74.375) -> (-87.6485, 74.375)
  line L8 (-87.6485, 74.375) -> (-87.6485, 73.125)
  constraints: 18 end point, 8 point on circle, 4 centre point
revolve "Revolution4" add sketch "Sketch_50" angle 90 about axis through (-87.6485, -122.3515, -74.375) along (0, 0, -1)
sketch "Sketch_51" plane through (0, -137.6485, 0) normal (0, 1, 0) x (1, 0, 0)
  line L0 (72.3515, 74.375) -> (72.3515, 73.125)
  line L1 (72.3515, 73.125) -> (71.3018, 73.125)
  arc A0 (70.0546, 73.7917) -> (71.3018, 73.125) centre (71.3018, 74.625) ccw
  line L2 (70.0546, 73.7917) -> (69.2528, 74.9917)
  arc A1 (69.2528, 74.9917) -> (69.0034, 75.125) centre (69.0034, 74.825) ccw
  line L3 (69.0034, 75.125) -> (64.5, 75.125)
  line L4 (64.5, 75.125) -> (64.5, 76.375)
  line L5 (64.5, 76.375) -> (69.0301, 76.375)
  arc A2 (70.2773, 75.7083) -> (69.0301, 76.375) centre (69.0301, 74.875) ccw
  line L6 (70.2773, 75.7083) -> (71.0791, 74.5083)
  arc A3 (71.0791, 74.5083) -> (71.3285, 74.375) centre (71.3285, 74.675) ccw
  line L7 (71.3285, 74.375) -> (72.3515, 74.375)
  line L8 (72.3515, 74.375) -> (72.3515, 73.125)
  constraints: 18 end point, 8 point on circle, 4 centre point
revolve "Revolution5" add sketch "Sketch_51" angle 90 about axis through (72.3515, -137.6485, -74.375) along (0, 0, 1)
sketch "Sketch_52" plane through (0, -137.6485, 0) normal (0, 1, 0) x (1, 0, 0)
  line L0 (-87.6485, 74.375) -> (-87.6485, 73.125)
  line L1 (-87.6485, 73.125) -> (-88.6982, 73.125)
  arc A0 (-89.9454, 73.7917) -> (-88.6982, 73.125) centre (-88.6982, 74.625) ccw
  line L2 (-89.9454, 73.7917) -> (-90.7472, 74.9917)
  arc A1 (-90.7472, 74.9917) -> (-90.9966, 75.125) centre (-90.9966, 74.825) ccw
  line L3 (-90.9966, 75.125) -> (-95.5, 75.125)
  line L4 (-95.5, 75.125) -> (-95.5, 76.375)
  line L5 (-95.5, 76.375) -> (-90.9699, 76.375)
  arc A2 (-89.7227, 75.7083) -> (-90.9699, 76.375) centre (-90.9699, 74.875) ccw
  line L6 (-89.7227, 75.7083) -> (-88.9209, 74.5083)
  arc A3 (-88.9209, 74.5083) -> (-88.6715, 74.375) centre (-88.6715, 74.675) ccw
  line L7 (-88.6715, 74.375) -> (-87.6485, 74.375)
  line L8 (-87.6485, 74.375) -> (-87.6485, 73.125)
  constraints: 18 end point, 8 point on circle, 4 centre point
revolve "Revolution6" add sketch "Sketch_52" angle 90 about axis through (-87.6485, -137.6485, -74.375) along (0, 0, 1)
sketch "Sketch_53" plane through (0, -137.6485, 0) normal (0, 1, 0) x (1, 0, 0)
  line L0 (87.6485, 73.125) -> (87.6485, 74.375)
  line L1 (87.6485, 74.375) -> (88.6715, 74.375)
  arc A0 (88.6715, 74.375) -> (88.9209, 74.5083) centre (88.6715, 74.675) ccw
  line L2 (88.9209, 74.5083) -> (89.7227, 75.7083)
  arc A1 (90.9699, 76.375) -> (89.7227, 75.7083) centre (90.9699, 74.875) ccw
  line L3 (90.9699, 76.375) -> (95.5, 76.375)
  line L4 (95.5, 76.375) -> (95.5, 75.125)
  line L5 (95.5, 75.125) -> (90.9966, 75.125)
  arc A2 (90.9966, 75.125) -> (90.7472, 74.9917) centre (90.9966, 74.825) ccw
  line L6 (90.7472, 74.9917) -> (89.9454, 73.7917)
  arc A3 (88.6982, 73.125) -> (89.9454, 73.7917) centre (88.6982, 74.625) ccw
  line L7 (88.6982, 73.125) -> (87.6485, 73.125)
  line L8 (87.6485, 73.125) -> (87.6485, 74.375)
  constraints: 18 end point, 8 point on circle, 4 centre point
revolve "Revolution7" add sketch "Sketch_53" angle 90 about axis through (87.6485, -137.6485, -73.125) along (0, 0, -1)
sketch "Sketch_54" plane through (0, -137.6485, 0) normal (0, 1, 0) x (1, 0, 0)
  line L0 (-72.3515, 73.125) -> (-72.3515, 74.375)
  line L1 (-72.3515, 74.375) -> (-71.3285, 74.375)
  arc A0 (-71.3285, 74.375) -> (-71.0791, 74.5083) centre (-71.3285, 74.675) ccw
  line L2 (-71.0791, 74.5083) -> (-70.2773, 75.7083)
  arc A1 (-69.0301, 76.375) -> (-70.2773, 75.7083) centre (-69.0301, 74.875) ccw
  line L3 (-69.0301, 76.375) -> (-64.5, 76.375)
  line L4 (-64.5, 76.375) -> (-64.5, 75.125)
  line L5 (-64.5, 75.125) -> (-69.0034, 75.125)
  arc A2 (-69.0034, 75.125) -> (-69.2528, 74.9917) centre (-69.0034, 74.825) ccw
  line L6 (-69.2528, 74.9917) -> (-70.0546, 73.7917)
  arc A3 (-71.3018, 73.125) -> (-70.0546, 73.7917) centre (-71.3018, 74.625) ccw
  line L7 (-71.3018, 73.125) -> (-72.3515, 73.125)
  line L8 (-72.3515, 73.125) -> (-72.3515, 74.375)
  constraints: 18 end point, 8 point on circle, 4 centre point
revolve "Revolution8" add sketch "Sketch_54" angle 90 about axis through (-72.3515, -137.6485, -73.125) along (0, 0, -1)
sketch "Sketch_55" plane through (0, 122.3515, 0) normal (0, 1, 0) x (1, 0, 0)
  line L0 (72.3515, 74.375) -> (72.3515, 73.125)
  line L1 (72.3515, 73.125) -> (71.3018, 73.125)
  arc A0 (70.0546, 73.7917) -> (71.3018, 73.125) centre (71.3018, 74.625) ccw
  line L2 (70.0546, 73.7917) -> (69.2528, 74.9917)
  arc A1 (69.2528, 74.9917) -> (69.0034, 75.125) centre (69.0034, 74.825) ccw
  line L3 (69.0034, 75.125) -> (64.5, 75.125)
  line L4 (64.5, 75.125) -> (64.5, 76.375)
  line L5 (64.5, 76.375) -> (69.0301, 76.375)
  arc A2 (70.2773, 75.7083) -> (69.0301, 76.375) centre (69.0301, 74.875) ccw
  line L6 (70.2773, 75.7083) -> (71.0791, 74.5083)
  arc A3 (71.0791, 74.5083) -> (71.3285, 74.375) centre (71.3285, 74.675) ccw
  line L7 (71.3285, 74.375) -> (72.3515, 74.375)
  line L8 (72.3515, 74.375) -> (72.3515, 73.125)
  constraints: 18 end point, 8 point on circle, 4 centre point
revolve "Revolution9" add sketch "Sketch_55" angle 90 about axis through (72.3515, 122.3515, -74.375) along (0, 0, 1)
sketch "Sketch_56" plane through (0, 122.3515, 0) normal (0, 1, 0) x (1, 0, 0)
  line L0 (-87.6485, 74.375) -> (-87.6485, 73.125)
  line L1 (-87.6485, 73.125) -> (-88.6982, 73.125)
  arc A0 (-89.9454, 73.7917) -> (-88.6982, 73.125) centre (-88.6982, 74.625) ccw
  line L2 (-89.9454, 73.7917) -> (-90.7472, 74.9917)
  arc A1 (-90.7472, 74.9917) -> (-90.9966, 75.125) centre (-90.9966, 74.825) ccw
  line L3 (-90.9966, 75.125) -> (-95.5, 75.125)
  line L4 (-95.5, 75.125) -> (-95.5, 76.375)
  line L5 (-95.5, 76.375) -> (-90.9699, 76.375)
  arc A2 (-89.7227, 75.7083) -> (-90.9699, 76.375) centre (-90.9699, 74.875) ccw
  line L6 (-89.7227, 75.7083) -> (-88.9209, 74.5083)
  arc A3 (-88.9209, 74.5083) -> (-88.6715, 74.375) centre (-88.6715, 74.675) ccw
  line L7 (-88.6715, 74.375) -> (-87.6485, 74.375)
  line L8 (-87.6485, 74.375) -> (-87.6485, 73.125)
  constraints: 18 end point, 8 point on circle, 4 centre point
revolve "Revolution10" add sketch "Sketch_56" angle 90 about axis through (-87.6485, 122.3515, -74.375) along (0, 0, 1)
sketch "Sketch_57" plane through (0, 122.3515, 0) normal (0, 1, 0) x (1, 0, 0)
  line L0 (87.6485, 73.125) -> (87.6485, 74.375)
  line L1 (87.6485, 74.375) -> (88.6715, 74.375)
  arc A0 (88.6715, 74.375) -> (88.9209, 74.5083) centre (88.6715, 74.675) ccw
  line L2 (88.9209, 74.5083) -> (89.7227, 75.7083)
  arc A1 (90.9699, 76.375) -> (89.7227, 75.7083) centre (90.9699, 74.875) ccw
  line L3 (90.9699, 76.375) -> (95.5, 76.375)
  line L4 (95.5, 76.375) -> (95.5, 75.125)
  line L5 (95.5, 75.125) -> (90.9966, 75.125)
  arc A2 (90.9966, 75.125) -> (90.7472, 74.9917) centre (90.9966, 74.825) ccw
  line L6 (90.7472, 74.9917) -> (89.9454, 73.7917)
  arc A3 (88.6982, 73.125) -> (89.9454, 73.7917) centre (88.6982, 74.625) ccw
  line L7 (88.6982, 73.125) -> (87.6485, 73.125)
  line L8 (87.6485, 73.125) -> (87.6485, 74.375)
  constraints: 18 end point, 8 point on circle, 4 centre point
revolve "Revolution11" add sketch "Sketch_57" angle 90 about axis through (87.6485, 122.3515, -73.125) along (0, 0, -1)
sketch "Sketch_58" plane through (0, 122.3515, 0) normal (0, 1, 0) x (1, 0, 0)
  line L0 (-72.3515, 73.125) -> (-72.3515, 74.375)
  line L1 (-72.3515, 74.375) -> (-71.3285, 74.375)
  arc A0 (-71.3285, 74.375) -> (-71.0791, 74.5083) centre (-71.3285, 74.675) ccw
  line L2 (-71.0791, 74.5083) -> (-70.2773, 75.7083)
  arc A1 (-69.0301, 76.375) -> (-70.2773, 75.7083) centre (-69.0301, 74.875) ccw
  line L3 (-69.0301, 76.375) -> (-64.5, 76.375)
  line L4 (-64.5, 76.375) -> (-64.5, 75.125)
  line L5 (-64.5, 75.125) -> (-69.0034, 75.125)
  arc A2 (-69.0034, 75.125) -> (-69.2528, 74.9917) centre (-69.0034, 74.825) ccw
  line L6 (-69.2528, 74.9917) -> (-70.0546, 73.7917)
  arc A3 (-71.3018, 73.125) -> (-70.0546, 73.7917) centre (-71.3018, 74.625) ccw
  line L7 (-71.3018, 73.125) -> (-72.3515, 73.125)
  line L8 (-72.3515, 73.125) -> (-72.3515, 74.375)
  constraints: 18 end point, 8 point on circle, 4 centre point
revolve "Revolution12" add sketch "Sketch_58" angle 90 about axis through (-72.3515, 122.3515, -73.125) along (0, 0, -1)
sketch "Sketch_59" plane through (0, 137.6485, 0) normal (0, 1, 0) x (1, 0, 0)
  line L0 (87.6485, 73.125) -> (87.6485, 74.375)
  line L1 (87.6485, 74.375) -> (88.6715, 74.375)
  arc A0 (88.6715, 74.375) -> (88.9209, 74.5083) centre (88.6715, 74.675) ccw
  line L2 (88.9209, 74.5083) -> (89.7227, 75.7083)
  arc A1 (90.9699, 76.375) -> (89.7227, 75.7083) centre (90.9699, 74.875) ccw
  line L3 (90.9699, 76.375) -> (95.5, 76.375)
  line L4 (95.5, 76.375) -> (95.5, 75.125)
  line L5 (95.5, 75.125) -> (90.9966, 75.125)
  arc A2 (90.9966, 75.125) -> (90.7472, 74.9917) centre (90.9966, 74.825) ccw
  line L6 (90.7472, 74.9917) -> (89.9454, 73.7917)
  arc A3 (88.6982, 73.125) -> (89.9454, 73.7917) centre (88.6982, 74.625) ccw
  line L7 (88.6982, 73.125) -> (87.6485, 73.125)
  line L8 (87.6485, 73.125) -> (87.6485, 74.375)
  constraints: 18 end point, 8 point on circle, 4 centre point
revolve "Revolution13" add sketch "Sketch_59" angle 90 about axis through (87.6485, 137.6485, -73.125) along (0, 0, 1)
sketch "Sketch_60" plane through (0, 137.6485, 0) normal (0, 1, 0) x (1, 0, 0)
  line L0 (-87.6485, 74.375) -> (-87.6485, 73.125)
  line L1 (-87.6485, 73.125) -> (-88.6982, 73.125)
  arc A0 (-89.9454, 73.7917) -> (-88.6982, 73.125) centre (-88.6982, 74.625) ccw
  line L2 (-89.9454, 73.7917) -> (-90.7472, 74.9917)
  arc A1 (-90.7472, 74.9917) -> (-90.9966, 75.125) centre (-90.9966, 74.825) ccw
  line L3 (-90.9966, 75.125) -> (-95.5, 75.125)
  line L4 (-95.5, 75.125) -> (-95.5, 76.375)
  line L5 (-95.5, 76.375) -> (-90.9699, 76.375)
  arc A2 (-89.7227, 75.7083) -> (-90.9699, 76.375) centre (-90.9699, 74.875) ccw
  line L6 (-89.7227, 75.7083) -> (-88.9209, 74.5083)
  arc A3 (-88.9209, 74.5083) -> (-88.6715, 74.375) centre (-88.6715, 74.675) ccw
  line L7 (-88.6715, 74.375) -> (-87.6485, 74.375)
  line L8 (-87.6485, 74.375) -> (-87.6485, 73.125)
  constraints: 18 end point, 8 point on circle, 4 centre point
revolve "Revolution14" add sketch "Sketch_60" angle 90 about axis through (-87.6485, 137.6485, -74.375) along (0, 0, -1)
sketch "Sketch_61" plane through (0, 137.6485, 0) normal (0, 1, 0) x (1, 0, 0)
  line L0 (-72.3515, 73.125) -> (-72.3515, 74.375)
  line L1 (-72.3515, 74.375) -> (-71.3285, 74.375)
  arc A0 (-71.3285, 74.375) -> (-71.0791, 74.5083) centre (-71.3285, 74.675) ccw
  line L2 (-71.0791, 74.5083) -> (-70.2773, 75.7083)
  arc A1 (-69.0301, 76.375) -> (-70.2773, 75.7083) centre (-69.0301, 74.875) ccw
  line L3 (-69.0301, 76.375) -> (-64.5, 76.375)
  line L4 (-64.5, 76.375) -> (-64.5, 75.125)
  line L5 (-64.5, 75.125) -> (-69.0034, 75.125)
  arc A2 (-69.0034, 75.125) -> (-69.2528, 74.9917) centre (-69.0034, 74.825) ccw
  line L6 (-69.2528, 74.9917) -> (-70.0546, 73.7917)
  arc A3 (-71.3018, 73.125) -> (-70.0546, 73.7917) centre (-71.3018, 74.625) ccw
  line L7 (-71.3018, 73.125) -> (-72.3515, 73.125)
  line L8 (-72.3515, 73.125) -> (-72.3515, 74.375)
  constraints: 18 end point, 8 point on circle, 4 centre point
revolve "Revolution15" add sketch "Sketch_61" angle 90 about axis through (-72.3515, 137.6485, -73.125) along (0, 0, 1)
sketch "Sketch_62" plane through (0, 137.6485, 0) normal (0, 1, 0) x (1, 0, 0)
  line L0 (72.3515, 74.375) -> (72.3515, 73.125)
  line L1 (72.3515, 73.125) -> (71.3018, 73.125)
  arc A0 (70.0546, 73.7917) -> (71.3018, 73.125) centre (71.3018, 74.625) ccw
  line L2 (70.0546, 73.7917) -> (69.2528, 74.9917)
  arc A1 (69.2528, 74.9917) -> (69.0034, 75.125) centre (69.0034, 74.825) ccw
  line L3 (69.0034, 75.125) -> (64.5, 75.125)
  line L4 (64.5, 75.125) -> (64.5, 76.375)
  line L5 (64.5, 76.375) -> (69.0301, 76.375)
  arc A2 (70.2773, 75.7083) -> (69.0301, 76.375) centre (69.0301, 74.875) ccw
  line L6 (70.2773, 75.7083) -> (71.0791, 74.5083)
  arc A3 (71.0791, 74.5083) -> (71.3285, 74.375) centre (71.3285, 74.675) ccw
  line L7 (71.3285, 74.375) -> (72.3515, 74.375)
  line L8 (72.3515, 74.375) -> (72.3515, 73.125)
  constraints: 18 end point, 8 point on circle, 4 centre point
revolve "Revolution16" add sketch "Sketch_62" angle 90 about axis through (72.3515, 137.6485, -74.375) along (0, 0, -1)
sketch "Sketch33" plane through (91.8, -141.8, 62.8605) normal (1, 0, 0) x (0, 0, -1)
  point P0 (-2.9845, 241.8)
hole "Hole1" at (91.8, 100, 65.845) direction (-1, 0, 0) diameter 3.2 depth 1.25
sketch "Sketch34" plane through (91.8, -141.8, 62.8605) normal (1, 0, 0) x (0, 0, -1)
  point P0 (-2.9845, 228.8)
hole "Hole2" at (91.8, 87, 65.845) direction (-1, 0, 0) diameter 3.2 depth 1.25
sketch "Sketch35" plane through (91.8, -141.8, 62.8605) normal (1, 0, 0) x (0, 0, -1)
  point P0 (-2.9845, 54.8)
hole "Hole3" at (91.8, -87, 65.845) direction (-1, 0, 0) diameter 3.2 depth 1.25
sketch "Sketch36" plane through (91.8, -141.8, 62.8605) normal (1, 0, 0) x (0, 0, -1)
  point P0 (-2.9845, 41.8)
hole "Hole4" at (91.8, -100, 65.845) direction (-1, 0, 0) diameter 3.2 depth 1.25
sketch "Sketch_75" plane through (0, 0, 65.845) normal (0, 0, 1) x (1, 0, 0)
  line L0 (96.05, 100) -> (88.4, 100)
  line L1 (88.4, 100) -> (88.4, 101.54)
  arc A0 (89.35, 102.6) -> (88.4, 101.54) centre (91.5789, 99.6467) ccw
  line L2 (89.35, 102.6) -> (89.35, 103.1)
  arc A1 (90.05, 103.1) -> (89.35, 103.1) centre (89.7, 103.1) ccw
  line L3 (90.05, 103.1) -> (90.05, 103.5)
  line L4 (90.05, 103.5) -> (90.55, 103.5)
  line L5 (90.55, 103.5) -> (90.55, 101.5)
  line L6 (90.55, 101.5) -> (95.7435, 101.5)
  line L7 (95.7435, 101.5) -> (96.05, 101.1935)
  line L8 (96.05, 101.1935) -> (96.05, 100)
  line L9 (96.05, 100) -> (88.4, 100)
  constraints: 20 end point, 4 point on circle, 2 centre point
revolve "Revolution17" add sketch "Sketch_75" angle 360 about axis through (96.05, 100, 65.845) along (1, 0, 0)
sketch "Sketch_76" plane through (0, 0, 65.845) normal (0, 0, 1) x (1, 0, 0)
  line L0 (96.05, 87) -> (88.4, 87)
  line L1 (88.4, 87) -> (88.4, 88.54)
  arc A0 (89.35, 89.6) -> (88.4, 88.54) centre (91.5789, 86.6467) ccw
  line L2 (89.35, 89.6) -> (89.35, 90.1)
  arc A1 (90.05, 90.1) -> (89.35, 90.1) centre (89.7, 90.1) ccw
  line L3 (90.05, 90.1) -> (90.05, 90.5)
  line L4 (90.05, 90.5) -> (90.55, 90.5)
  line L5 (90.55, 90.5) -> (90.55, 88.5)
  line L6 (90.55, 88.5) -> (95.7435, 88.5)
  line L7 (95.7435, 88.5) -> (96.05, 88.1935)
  line L8 (96.05, 88.1935) -> (96.05, 87)
  line L9 (96.05, 87) -> (88.4, 87)
  constraints: 20 end point, 4 point on circle, 2 centre point
revolve "Revolution18" add sketch "Sketch_76" angle 360 about axis through (96.05, 87, 65.845) along (1, 0, 0)
sketch "Sketch_77" plane through (0, 0, 65.845) normal (0, 0, 1) x (1, 0, 0)
  line L0 (96.05, -87) -> (88.4, -87)
  line L1 (88.4, -87) -> (88.4, -85.46)
  arc A0 (89.35, -84.4) -> (88.4, -85.46) centre (91.5789, -87.3533) ccw
  line L2 (89.35, -84.4) -> (89.35, -83.9)
  arc A1 (90.05, -83.9) -> (89.35, -83.9) centre (89.7, -83.9) ccw
  line L3 (90.05, -83.9) -> (90.05, -83.5)
  line L4 (90.05, -83.5) -> (90.55, -83.5)
  line L5 (90.55, -83.5) -> (90.55, -85.5)
  line L6 (90.55, -85.5) -> (95.7435, -85.5)
  line L7 (95.7435, -85.5) -> (96.05, -85.8065)
  line L8 (96.05, -85.8065) -> (96.05, -87)
  line L9 (96.05, -87) -> (88.4, -87)
  constraints: 20 end point, 4 point on circle, 2 centre point
revolve "Revolution19" add sketch "Sketch_77" angle 360 about axis through (96.05, -87, 65.845) along (1, 0, 0)
sketch "Sketch_78" plane through (0, 0, 65.845) normal (0, 0, 1) x (1, 0, 0)
  line L0 (96.05, -100) -> (88.4, -100)
  line L1 (88.4, -100) -> (88.4, -98.46)
  arc A0 (89.35, -97.4) -> (88.4, -98.46) centre (91.5789, -100.3533) ccw
  line L2 (89.35, -97.4) -> (89.35, -96.9)
  arc A1 (90.05, -96.9) -> (89.35, -96.9) centre (89.7, -96.9) ccw
  line L3 (90.05, -96.9) -> (90.05, -96.5)
  line L4 (90.05, -96.5) -> (90.55, -96.5)
  line L5 (90.55, -96.5) -> (90.55, -98.5)
  line L6 (90.55, -98.5) -> (95.7435, -98.5)
  line L7 (95.7435, -98.5) -> (96.05, -98.8065)
  line L8 (96.05, -98.8065) -> (96.05, -100)
  line L9 (96.05, -100) -> (88.4, -100)
  constraints: 20 end point, 4 point on circle, 2 centre point
revolve "Revolution20" add sketch "Sketch_78" angle 360 about axis through (96.05, -100, 65.845) along (1, 0, 0)
sketch "Sketch_79" plane through (88.4, 0, 0) normal (1, 0, 0) x (0, 0, -1)
  arc A0 (-67.0296, 100.2724) -> (-67.0296, 99.7276) centre (-66.965, 100) ccw
  arc A1 (-66.6732, 99.1103) -> (-67.0296, 99.7276) centre (-67.1427, 99.2508) ccw
  arc A2 (-66.6732, 99.1103) -> (-66.2014, 98.8379) centre (-66.405, 99.0301) ccw
  arc A3 (-65.4886, 98.8379) -> (-66.2014, 98.8379) centre (-65.845, 98.5016) ccw
  arc A4 (-65.4886, 98.8379) -> (-65.0168, 99.1103) centre (-65.285, 99.0301) ccw
  arc A5 (-64.6604, 99.7276) -> (-65.0168, 99.1103) centre (-64.5473, 99.2508) ccw
  arc A6 (-64.6604, 99.7276) -> (-64.6604, 100.2724) centre (-64.725, 100) ccw
  arc A7 (-65.0168, 100.8897) -> (-64.6604, 100.2724) centre (-64.5473, 100.7492) ccw
  arc A8 (-65.0168, 100.8897) -> (-65.4886, 101.1621) centre (-65.285, 100.9699) ccw
  arc A9 (-66.2014, 101.1621) -> (-65.4886, 101.1621) centre (-65.845, 101.4984) ccw
  arc A10 (-66.2014, 101.1621) -> (-66.6732, 100.8897) centre (-66.405, 100.9699) ccw
  arc A11 (-67.0296, 100.2724) -> (-66.6732, 100.8897) centre (-67.1427, 100.7492) ccw
  constraints: 24 point on circle, 12 centre point
extrude "Extrusion17" cut sketch "Sketch_79" along normal blind 1.2
sketch "Sketch_80" plane through (88.4, 0, 0) normal (1, 0, 0) x (0, 0, -1)
  arc A0 (-67.0296, 87.2724) -> (-67.0296, 86.7276) centre (-66.965, 87) ccw
  arc A1 (-66.6732, 86.1103) -> (-67.0296, 86.7276) centre (-67.1427, 86.2508) ccw
  arc A2 (-66.6732, 86.1103) -> (-66.2014, 85.8379) centre (-66.405, 86.0301) ccw
  arc A3 (-65.4886, 85.8379) -> (-66.2014, 85.8379) centre (-65.845, 85.5016) ccw
  arc A4 (-65.4886, 85.8379) -> (-65.0168, 86.1103) centre (-65.285, 86.0301) ccw
  arc A5 (-64.6604, 86.7276) -> (-65.0168, 86.1103) centre (-64.5473, 86.2508) ccw
  arc A6 (-64.6604, 86.7276) -> (-64.6604, 87.2724) centre (-64.725, 87) ccw
  arc A7 (-65.0168, 87.8897) -> (-64.6604, 87.2724) centre (-64.5473, 87.7492) ccw
  arc A8 (-65.0168, 87.8897) -> (-65.4886, 88.1621) centre (-65.285, 87.9699) ccw
  arc A9 (-66.2014, 88.1621) -> (-65.4886, 88.1621) centre (-65.845, 88.4984) ccw
  arc A10 (-66.2014, 88.1621) -> (-66.6732, 87.8897) centre (-66.405, 87.9699) ccw
  arc A11 (-67.0296, 87.2724) -> (-66.6732, 87.8897) centre (-67.1427, 87.7492) ccw
  constraints: 24 point on circle, 12 centre point
extrude "Extrusion18" cut sketch "Sketch_80" along normal blind 1.2
sketch "Sketch_81" plane through (88.4, 0, 0) normal (1, 0, 0) x (0, 0, -1)
  arc A0 (-67.0296, -86.7276) -> (-67.0296, -87.2724) centre (-66.965, -87) ccw
  arc A1 (-66.6732, -87.8897) -> (-67.0296, -87.2724) centre (-67.1427, -87.7492) ccw
  arc A2 (-66.6732, -87.8897) -> (-66.2014, -88.1621) centre (-66.405, -87.9699) ccw
  arc A3 (-65.4886, -88.1621) -> (-66.2014, -88.1621) centre (-65.845, -88.4984) ccw
  arc A4 (-65.4886, -88.1621) -> (-65.0168, -87.8897) centre (-65.285, -87.9699) ccw
  arc A5 (-64.6604, -87.2724) -> (-65.0168, -87.8897) centre (-64.5473, -87.7492) ccw
  arc A6 (-64.6604, -87.2724) -> (-64.6604, -86.7276) centre (-64.725, -87) ccw
  arc A7 (-65.0168, -86.1103) -> (-64.6604, -86.7276) centre (-64.5473, -86.2508) ccw
  arc A8 (-65.0168, -86.1103) -> (-65.4886, -85.8379) centre (-65.285, -86.0301) ccw
  arc A9 (-66.2014, -85.8379) -> (-65.4886, -85.8379) centre (-65.845, -85.5016) ccw
  arc A10 (-66.2014, -85.8379) -> (-66.6732, -86.1103) centre (-66.405, -86.0301) ccw
  arc A11 (-67.0296, -86.7276) -> (-66.6732, -86.1103) centre (-67.1427, -86.2508) ccw
  constraints: 24 point on circle, 12 centre point
extrude "Extrusion19" cut sketch "Sketch_81" along normal blind 1.2
sketch "Sketch_82" plane through (88.4, 0, 0) normal (1, 0, 0) x (0, 0, -1)
  arc A0 (-67.0296, -99.7276) -> (-67.0296, -100.2724) centre (-66.965, -100) ccw
  arc A1 (-66.6732, -100.8897) -> (-67.0296, -100.2724) centre (-67.1427, -100.7492) ccw
  arc A2 (-66.6732, -100.8897) -> (-66.2014, -101.1621) centre (-66.405, -100.9699) ccw
  arc A3 (-65.4886, -101.1621) -> (-66.2014, -101.1621) centre (-65.845, -101.4984) ccw
  arc A4 (-65.4886, -101.1621) -> (-65.0168, -100.8897) centre (-65.285, -100.9699) ccw
  arc A5 (-64.6604, -100.2724) -> (-65.0168, -100.8897) centre (-64.5473, -100.7492) ccw
  arc A6 (-64.6604, -100.2724) -> (-64.6604, -99.7276) centre (-64.725, -100) ccw
  arc A7 (-65.0168, -99.1103) -> (-64.6604, -99.7276) centre (-64.5473, -99.2508) ccw
  arc A8 (-65.0168, -99.1103) -> (-65.4886, -98.8379) centre (-65.285, -99.0301) ccw
  arc A9 (-66.2014, -98.8379) -> (-65.4886, -98.8379) centre (-65.845, -98.5016) ccw
  arc A10 (-66.2014, -98.8379) -> (-66.6732, -99.1103) centre (-66.405, -99.0301) ccw
  arc A11 (-67.0296, -99.7276) -> (-66.6732, -99.1103) centre (-67.1427, -99.2508) ccw
  constraints: 24 point on circle, 12 centre point
extrude "Extrusion20" cut sketch "Sketch_82" along normal blind 1.2
ref_plane "GEHAEUSE_XY" through (0, 0, -76.375) normal (0, -1, 0) x (1, 0, 0)
ref_plane "GEHAEUSE_YZ" through (0, 0, -76.375) normal (1, 0, 0) x (0, 0, 1)
ref_plane "GEHAEUSE_ZX" through (0, 0, -76.375) normal (0, 0, 1) x (0, -1, 0)
ref_plane "to_HINGE_1_XY" through (91.75, 93.5, 65.845) normal (0, 1, 0) x (1, 0, 0)
ref_plane "to_HINGE_1_YZ" through (91.75, 93.5, 65.845) normal (1, 0, 0) x (0, 0, -1)
ref_plane "to_HINGE_1_ZX" through (91.75, 93.5, 65.845) normal (0, 0, -1) x (0, 1, 0)
ref_plane "to_HINGE_2_XY" through (91.75, -93.5, 65.845) normal (0, 1, 0) x (1, 0, 0)
ref_plane "to_HINGE_2_YZ" through (91.75, -93.5, 65.845) normal (1, 0, 0) x (0, 0, -1)
ref_plane "to_HINGE_2_ZX" through (91.75, -93.5, 65.845) normal (0, 0, -1) x (0, 1, 0)
ref_plane "to_L_Winkel_XY" through (98.75, 0, -61.025) normal (1, 0, 0) x (0, 0, -1)
ref_plane "to_L_Winkel_YZ" through (98.75, 0, -61.025) normal (0, 0, -1) x (0, 1, 0)
ref_plane "to_L_Winkel_ZX" through (98.75, 0, -61.025) normal (0, 1, 0) x (1, 0, 0)
ref_plane "to_L_Winkel_Bottom_XY" through (0, -148.75, -61.125) normal (0, -1, 0) x (1, 0, 0)
ref_plane "to_L_Winkel_Bottom_YZ" through (0, -148.75, -61.125) normal (1, 0, 0) x (0, 0, 1)
ref_plane "to_L_Winkel_Bottom_ZX" through (0, -148.75, -61.125) normal (0, 0, 1) x (0, -1, 0)
ref_plane "to_L_Winkel_Top_XY" through (0, 148.75, -61.125) normal (0, 1, 0) x (1, 0, 0)
ref_plane "to_L_Winkel_Top_YZ" through (0, 148.75, -61.125) normal (1, 0, 0) x (0, 0, -1)
ref_plane "to_L_Winkel_Top_ZX" through (0, 148.75, -61.125) normal (0, 0, -1) x (0, 1, 0)
ref_plane "to_L_Winkel_1_XY" through (-98.75, 0, -61.025) normal (-1, 0, 0) x (0, 0, -1)